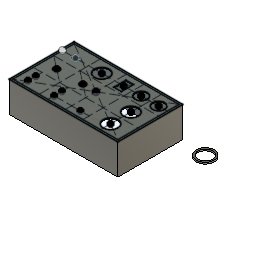
Panel 1 mini lite (hub) (Autodesk Fusion 360 design; units mm, degrees)
Autodesk Fusion 360 part; units mm, degrees
sketch "Sketch1" plane through (0, 0, 0) normal (0, 0, 1) x (1, 0, 0)
  line L0 (60, 35) -> (-60, 35)
  line L1 (-60, 35) -> (-60, -35)
  line L2 (-60, -35) -> (60, -35)
  line L3 (60, -35) -> (60, 35)
  line L4 (60, 35) -> (-60, -35) construction
  line L5 (-60, 35) -> (60, -35) construction
  line L6 (-30, 35) -> (-30, -35) construction
  line L7 (0, 35) -> (0, -35) construction
  line L8 (20, 35) -> (20, -35) construction
  line L9 (-60, 11.6667) -> (60, 11.6667) construction
  line L10 (-60, -11.6667) -> (60, -11.6667) construction
  line L11 (-60, 21.6667) -> (-30, 21.6667) construction
  circle A0 centre (-45, 21.6667) radius 3.2
  line L12 (-30, 21.6667) -> (0, 21.6667) construction
  circle A1 centre (-15, 21.6667) radius 8.25
  line L13 (20, 21.6667) -> (40, 21.6667) construction
  line L14 (40, 21.6667) -> (60, 21.6667) construction
  circle A2 centre (30, 21.6667) radius 6.75
  circle A3 centre (50, 21.6667) radius 6.75
  line L15 (-60, 11.6667) -> (-30, -11.6667) construction
  line L16 (-30, 11.6667) -> (0, -11.6667) construction
  circle A4 centre (-45, 0) radius 3.2
  circle A5 centre (-15, 0) radius 3.2
  line L17 (-50, -29.6222) -> (-50, -35) construction
  circle A6 centre (-50, -18.8444) radius 1.8
  circle A7 centre (-50, -27.8222) radius 1.8
  line L18 (-50, -11.6667) -> (-50, -17.0444) construction
  line L19 (-50, -17.0444) -> (-50, -20.6444) construction
  line L20 (-50, -20.6444) -> (-50, -26.0222) construction
  line L21 (-50, -26.0222) -> (-50, -29.1667) construction
  line L22 (-50, -29.1667) -> (-50, -29.6222) construction
  line L23 (-20, -29.6222) -> (-20, -35) construction
  circle A8 centre (-20, -18.8444) radius 1.8
  circle A9 centre (-20, -27.8222) radius 1.8
  line L24 (-20, -11.6667) -> (-20, -17.0444) construction
  line L25 (-20, -17.0444) -> (-20, -20.6444) construction
  line L26 (-20, -20.6444) -> (-20, -26.0222) construction
  line L27 (-20, -26.0222) -> (-20, -29.6222) construction
  line L28 (-20, -27.8222) -> (0, -27.8222) construction
  line L29 (0, -27.8222) -> (20, -27.8222) construction
  circle A10 centre (10, -27.8222) radius 1.8
  line L30 (40, 35) -> (40, 11.6667) construction
  line L31 (40, -11.6667) -> (40, -35) construction
  circle A11 centre (40, -23.3333) radius 8.25
  line L32 (40, 11.6667) -> (40, -11.6667) construction
  circle A12 centre (40, 0) radius 8.25
  line L33 (0, 21.6667) -> (20, 21.6667) construction
  line L34 (14.4, 28.6667) -> (5.6, 28.6667)
  line L35 (5.6, 28.6667) -> (5.6, 14.6667)
  line L36 (5.6, 14.6667) -> (14.4, 14.6667)
  line L37 (14.4, 14.6667) -> (14.4, 28.6667)
  line L38 (14.4, 28.6667) -> (5.6, 14.6667) construction
  line L39 (5.6, 28.6667) -> (14.4, 14.6667) construction
  line L40 (62, -37) -> (62, 37)
  line L41 (62, 37) -> (-62, 37)
  line L42 (-62, 37) -> (-62, -37)
  line L43 (-62, -37) -> (62, -37)
  point P0 (10, 21.6667)
  dimension "d1" = 120
  dimension "d2" = 70
  dimension "d6" = 30
  dimension "d7" = 30
  dimension "d8" = 20
  dimension "d9" = 20
  dimension "d10" = 23.3333
  dimension "d11" = 23.3333
  dimension "d12" = 23.3333
  dimension "d13" = 20
  dimension "d14" = 10
  dimension "d15" = 6.4
  dimension "d16" = 10
  dimension "d17" = 16.5
  dimension "d18" = 10
  dimension "d19" = 13.5
  dimension "d20" = 13.5
  dimension "d21" = 6.4
  dimension "d22" = 6.4
  dimension "d23" = 10
  dimension "d24" = 3.6
  dimension "d25" = 3.6
  dimension "d26" = 10
  dimension "d27" = 3.6
  dimension "d28" = 3.6
  dimension "d29" = 3.6
  dimension "d30" = 16.5
  dimension "d31" = 16.5
  dimension "d32" = 8.8
  dimension "d33" = 14
  dimension "d34" = 2
  constraint horizontal L0
  constraint perpendicular L0 L1
  constraint parallel L0 L2
  constraint parallel L1 L3
  constraint coincident L4 origin
  constraint coincident L5 origin
  constraint coincident L0 L6.start
  constraint coincident L2 L6.end
  constraint perpendicular L2 L6
  constraint coincident L0 L7.start
  constraint coincident L2 L7.end
  constraint perpendicular L2 L7
  constraint coincident L0 L8.start
  constraint coincident L2 L8.end
  constraint perpendicular L2 L8
  constraint coincident L0 L30.start
  constraint perpendicular L2 L30
  constraint coincident L1 L9.start
  constraint coincident L3 L9.end
  constraint perpendicular L3 L9
  constraint coincident L1 L10.start
  constraint coincident L3 L10.end
  constraint perpendicular L3 L10
  constraint coincident L6 L11.end
  constraint perpendicular L6 L11
  constraint midpoint L11 A0.centre
  constraint coincident L7 L12.end
  constraint horizontal L12
  constraint midpoint L12 A1.centre
  constraint coincident L8 L13.start
  constraint coincident L3 L14.end
  constraint perpendicular L3 L13
  constraint coincident L13.end L30
  constraint perpendicular L3 L14
  constraint midpoint L13 A2.centre
  constraint midpoint L14 A3.centre
  constraint coincident L6 L15.end
  constraint coincident L10 L15.end
  constraint coincident L6 L16.start
  constraint coincident L9 L16.start
  constraint midpoint L10 L16.end
  constraint midpoint L15 A4.centre
  constraint midpoint L16 A5.centre
  constraint coincident L10 L18.start
  constraint coincident L2 L17.end
  constraint perpendicular L2 L17
  constraint coincident L17 A6.centre
  constraint coincident L17 A7.centre
  constraint coincident A6 L18.end
  constraint perpendicular L2 L18
  constraint coincident A6 L19.end
  constraint perpendicular L2 L19
  constraint coincident A7 L20.end
  constraint perpendicular L2 L20
  constraint coincident L4 L21.end
  constraint perpendicular L2 L21
  constraint coincident A7 L17.start
  constraint perpendicular L2 L22
  constraint equal L18 L20
  constraint equal L17 L20
  constraint coincident L10 L24.start
  constraint coincident L2 L23.end
  constraint perpendicular L2 L23
  constraint coincident L23 A8.centre
  constraint coincident L23 A9.centre
  constraint coincident A8 L24.end
  constraint perpendicular L2 L24
  constraint coincident A8 L25.end
  constraint perpendicular L2 L25
  constraint coincident A9 L26.end
  constraint perpendicular L2 L26
  constraint coincident A9 L23.start
  constraint perpendicular L2 L27
  constraint equal L24 L26
  constraint equal L23 L26
  constraint coincident A9.centre L28.start
  constraint coincident L8 L29.end
  constraint perpendicular L8 L28
  constraint coincident L7 L28.end
  constraint perpendicular L8 L29
  constraint midpoint L29 A10.centre
  constraint coincident L10 L31.start
  constraint perpendicular L10 L31
  constraint coincident L31 A11.centre
  constraint midpoint L31 A11.centre
  constraint coincident L2 L31.end
  constraint coincident L9 L30.end
  constraint perpendicular L2 L32
  constraint midpoint L32 A12.centre
  constraint horizontal L34
  constraint perpendicular L34 L35
  constraint parallel L34 L36
  constraint parallel L35 L37
  constraint coincident L38 P0
  constraint coincident L39 P0
  constraint midpoint L33 P0
  measures "d1" distance of L1.end L2.end
  measures "d2" distance of L0.end L1.end
  measures "d6" distance of L1 L6
  measures "d7" distance of L6 L7
  measures "d8" distance of L7 L8
  measures "d9" distance of L8 L30
  measures "d10" distance of L0 L9
  measures "d11" distance of L9 L10
  measures "d12" distance of L2 L10
  measures "d13" distance of L3 L30
  measures "d14" distance of L9 L11
  measures "d15" diameter of A0
  measures "d16" distance of L9 L12
  measures "d17" diameter of A1
  measures "d18" distance of L9 L13
  measures "d19" diameter of A2
  measures "d20" diameter of A3
  measures "d21" diameter of A4
  measures "d22" diameter of A5
  measures "d23" distance of L1 L17
  measures "d24" diameter of A6
  measures "d25" diameter of A7
  measures "d26" distance of L6 L23
  measures "d27" diameter of A8
  measures "d28" diameter of A9
  measures "d29" diameter of A10
  measures "d30" diameter of A11
  measures "d31" diameter of A12
  measures "d32" distance of L35.end L36.end
  measures "d33" distance of L34.end L35.end
extrude "Extrude1" add sketch "Sketch1" against normal blind 1 contours L0 L1 L2 L3 makes body 1
extrude "Extrude2" add sketch "Sketch1" against normal blind 35 contours L40 L41 L42 L43 bodies 1
sketch "Sketch2" plane through (0, 0, 0) normal (0, 0, 1) x (1, 0, 0)
  circle A0 centre (125, 0) radius 8.25
  circle A1 centre (125, 0) radius 10.25
  dimension "d39" = 16.5
  dimension "d40" = 2
  measures "d39" diameter of A0
extrude "Extrude3" add sketch "Sketch2" along normal blind 1.8 separate body makes body 2
move_body "Move1" bodies 2 to x (1, 0, 0) y (0, 1, 0) z (0, 0, 1) at (0, 0, -1.8)
equation "d10 = ( 70 / 3 ) * 1 mm"
equation "d11 = ( 70 / 3 ) * 1 mm"
equation "d35 = -mm"
